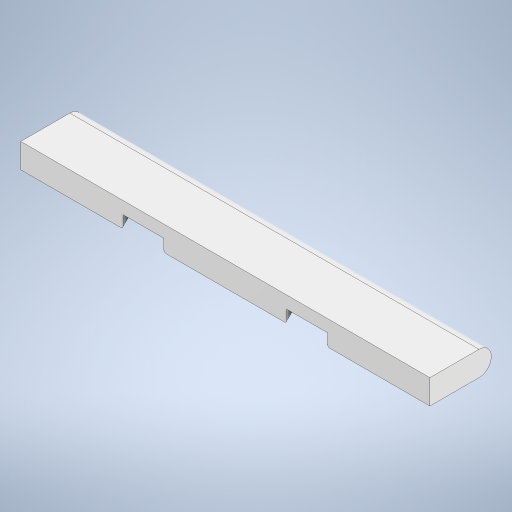
# Autodesk Inventor part: Test2
Saved by Autodesk Inventor 2023.1 (Build 271208000, 208)
## iProperties
Created: 2023-02-07
Part Number: Test2
Material: ABS Plastic
Document SubType Name: Modeling
Designer: 19644
Density: 1.06 g/cm^3
Appearance: Smooth - White
Author: 19644
## iProperties of the stored document Test2_3DPrint.ipt
Created: 2023-02-07
Part Number: Test2_3DPrint
Material: Generic
Document SubType Name: Modeling
Designer: 19644
Density: 1 g/cm^3
Appearance: Default
Author: 19644
Autodesk Inventor part; units mm, degrees
ref_plane "YZ Plane" through (0, 0, 0) normal (1, 0, 0) x (0, 1, 0)
ref_plane "XZ Plane" through (0, 0, 0) normal (0, 1, 0) x (-1, 0, 0)
ref_plane "XY Plane" through (0, 0, 0) normal (0, 0, 1) x (1, 0, 0)
sketch "Sketch1" plane through (0, 0, 0) normal (0, 1, 0) x (-1, 0, 0)
  line L0 (100, -50) -> (-100, -50)
  line L1 (-100, -50) -> (-100, 50)
  line L2 (-100, 50) -> (100, 50)
  line L3 (100, 50) -> (100, -50)
  line L4 (100, -50) -> (-100, 50) construction
  line L5 (-100, -50) -> (100, 50) construction
  line L6 (-40, -30) -> (-80, -30)
  line L7 (-50, -50) -> (-70, -50)
  line L8 (-40, -30) -> (-50, -50)
  line L9 (-80, -30) -> (-70, -50)
  line L10 (80, -30) -> (40, -30)
  line L11 (70, -50) -> (50, -50)
  line L12 (80, -30) -> (70, -50)
  line L13 (40, -30) -> (50, -50)
  line L14 (-100, -10) -> (-100, 10)
  line L15 (-80, -20) -> (-80, 20)
  line L16 (-80, -20) -> (-100, -10)
  line L17 (-80, 20) -> (-100, 10)
  line L18 (100, -50) -> (-100, -50)
  line L19 (-100, -50) -> (-100, -80)
  line L20 (-100, -80) -> (100, -80)
  line L21 (100, -80) -> (100, -50)
  line L22 (-40, -70) -> (-80, -70)
  line L23 (-40, -70) -> (-50, -50)
  line L24 (-80, -70) -> (-70, -50)
  line L25 (80, -70) -> (40, -70)
  line L26 (80, -70) -> (70, -50)
  line L27 (40, -70) -> (50, -50)
  line L28 (-100, -80) -> (-200, -80)
  line L29 (-200, -80) -> (-200, -50)
  line L30 (-200, -50) -> (-100, -50)
  line L31 (-100, -50) -> (-100, -80)
  line L32 (-160, -70) -> (-150, -50)
  line L33 (-160, -70) -> (-120, -70)
  line L34 (-120, -70) -> (-130, -50)
  line L35 (0, -80) -> (0, -50)
  point P0 (0, 0)
  point P1 (-100, 10)
  point P2 (-100, -10)
  point P3 (-70, -50)
  point P4 (-50, -50)
  point P5 (70, -50)
  point P6 (0, 0)
  point P7 (0, 0)
  point P8 (-100, -50)
  point P9 (-100, -50)
  point P10 (-100, -50)
  dimension "d72" = 200
  dimension "d73" = 100
  dimension "d78" = 20
  dimension "d79" = 40
  dimension "d80" = 20
  dimension "d81" = 10
  dimension "d82" = 20
  dimension "d83" = 40
  dimension "d84" = 20
  dimension "d85" = 10
  dimension "d86" = 120
  dimension "d87" = 30
  dimension "d88" = 0
  dimension "d89" = 0
  dimension "d90" = 40
  dimension "d91" = 20
  dimension "d92" = 20
  dimension "d93" = 10
  dimension "d94" = 40
  dimension "d95" = 0
  dimension "d114" = 200
  dimension "d115" = 30
  dimension "d128" = 100
  constraints: 72 end point, 8 symmetric about line, 7 horizontal, 6 parallel, 5 midpoint, 3 perpendicular, 2 vertical, 1 coincident
  measures "d72" distance of L1.end L2.end
  measures "d73" distance of L0.end L1.end
  measures "d78" distance of L7.start L7.end
  measures "d79" distance of L6.start L6.end
  measures "d80" distance from line of L7.end L6
  measures "d81" horizontal distance of L6.end L7.end
  measures "d82" distance of L11.start L11.end
  measures "d83" distance of L10.start L10.end
  measures "d84" distance from line of L11.end L10
  measures "d85" horizontal distance of L10.end L11.end
  measures "d86" distance of L7.end L11.end
  measures "d87" distance from line of L3 L11.start
  measures "d88" distance between parallel lines of L0 L7
  measures "d89" distance between parallel lines of L0 L11
  measures "d90" distance of L15.start L15.end
  measures "d91" distance of L14.start L14.end
  measures "d92" distance between parallel lines of L14 L15
  measures "d93" vertical distance of L15.start L14.start
  measures "d94" distance from line of L0 L14.start
  measures "d95" distance between parallel lines of L1 L14
  measures "d114" distance of L20.end L19.end
  measures "d115" distance of L19.end L18.end
  measures "d128" distance of L29.end L30.end
sketch "Sketch1 outline for Extrusion28" plane through (0, 0, 0) normal (0, 1, 0) x (-1, 0, 0)
  line L0 (-200, -50) -> (-200, -80)
  line L1 (-100, -50) -> (-200, -50)
  line L2 (-100, -80) -> (-100, -50)
  line L3 (-200, -80) -> (-100, -80)
extrude "Extrusion28" add sketch "Sketch1 outline for Extrusion28" along normal blind 12
sketch "Sketch1 outline for Extrusion29" plane through (0, 0, 0) normal (0, 1, 0) x (-1, 0, 0)
  line L0 (-160, -70) -> (-120, -70)
  line L1 (-150, -50) -> (-160, -70)
  line L2 (-130, -50) -> (-150, -50)
  line L3 (-120, -70) -> (-130, -50)
extrude "Extrusion29" cut sketch "Sketch1 outline for Extrusion29" along normal blind 6
fillet "Fillet17" radius 6 2 edges at (150, 0, -80) (150, 12, -80)
fillet "Fillet18" radius 2 2 edges at (120, 3, -70) (160, 3, -70)
fillet "Fillet19" radius 1 5 edges at (158.4652, 0, -69.0515) (140, 0, -70) (121.5348, 0, -69.0515) (125.7236, 0, -58.5528) (154.2764, 0, -58.5528)
mirror "Mirror1" about plane through (100, 0, -80) normal (-1, 0, 0) of "Extrusion28", "Fillet17", "Extrusion29", "Fillet18", "Fillet19"
body "Solid12"
